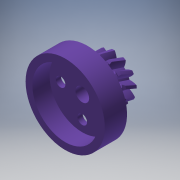
# Autodesk Inventor part: Stirnzahnrad2
Saved by Autodesk Inventor 2019.1 (Build 231200000, 200)
## iProperties
Created: 2019-01-01
Part Number: Stirnzahnrad2
Material: Steel
Document SubType Name: Modeling
Designer: JochenAlt
Categories: <?xml version="1.0" encoding="UTF-16"?> <MemberInstance><Categories><FamilyTemplate><FamilyTemplateParameter ValueType="xs:double" Id="1" ObjectReferenceKey="da_z" ObjectType="kUserParameterObject"/><FamilyTemplateParameter ValueType="xs:double" Id="2" ObjectReferenceKey="da_b" ObjectType="kUserParameterObject"/><FamilyTemplateParameter ValueType="xs:double" Id="3" ObjectReferenceKey="da_beta" ObjectType="kUserParameterObject"/><FamilyTemplateParameter ValueType="xs:double" Id="4" ObjectReferenceKey="da_da" ObjectType="kUserParameterObject"/><FamilyTemplateParameter ValueType="xs:double" Id="5" ObjectReferenceKey="da_aw" ObjectType="kUserParameterObject"/></FamilyTemplate><ParamToTemplateMap><ParamToTemplate CategoryParameter="//CategoryParameter[@InternalName='046C89C9-8512-4d59-83FE-43B91F4F132A']" TemplateParameter="1"/><ParamToTemplate CategoryParameter="//CategoryParameter[@InternalName='2552DF32-E462-4b46-AEBF-C6C7768E72AC']" TemplateParameter="2"/><ParamToTemplate CategoryParameter="//CategoryParameter[@InternalName='C9EE641D-15FC-4fae-A226-E94C4372FDD7']" TemplateParameter="3"/><ParamToTemplate><ParamToTemplate CategoryParameter="//CategoryParameter[@InternalName='00B6519A-459B-49c7-AD84-2E56D39A5744']" ConstantValue="-0.200000"/></ParamToTemplate><ParamToTemplate><ParamToTemplate CategoryParameter="//CategoryParameter[@InternalName='04B31F0E-C7A6-4894-AA32-9629BEFACF47']" ConstantValue="1.000000"/></ParamToTemplate><ParamToTemplate><ParamToTemplate CategoryParameter="//CategoryParameter[@InternalName='43CBEC2E-7847-49e7-A936-2F7889FCB2D9']" ConstantValue="0.250000"/></ParamToTemplate><ParamToTemplate><ParamToTemplate CategoryParameter="//CategoryParameter[@InternalName='B1EFC894-105D-4ebd-86BF-FA20ED196853']" ConstantValue="0.350000"/></ParamToTemplate><ParamToTemplate><ParamToTemplate CategoryParameter="//CategoryParameter[@InternalName='51175063-3D10-4879-93E8-6246FE8B403D']" ConstantValue="2060000000.000000"/></ParamToTemplate><ParamToTemplate><ParamToTemplate CategoryParameter="//CategoryParameter[@InternalName='A3A52E27-4454-46a9-B0BD-C932399B70AF']" ConstantValue="0.300000"/></ParamToTemplate><ParamToTemplate><ParamToTemplate CategoryParameter="//CategoryParameter[@InternalName='91B76062-C214-41d9-B1B9-14D2AB99603D']" ConstantValue="0.090000"/></ParamToTemplate><ParamToTemplate><ParamToTemplate CategoryParameter="//CategoryParameter[@InternalName='374E806E-8B8A-4dda-A9AA-1039D6500AD2']" ConstantValue="11.111111"/></ParamToTemplate><ParamToTemplate><ParamToTemplate CategoryParameter="//CategoryParameter[@InternalName='2D373A89-B862-43d6-8D0B-0CBF12AB9F6C']" ConstantValue="0.349066"/></ParamToTemplate><ParamToTemplate CategoryParameter="//CategoryParameter[@InternalName='37777632-D6A2-4fac-9D53-DB8ACD95C989']" TemplateParameter="4"/><ParamToTemplate CategoryParameter="//CategoryParameter[@InternalName='FD1017F1-B727-4f7e-9707-0F86F1FF9423']" TemplateParameter="5"/><ParamToTemplate><ParamToTemplate CategoryParameter="//CategoryParameter[@InternalName='9E1B4470-B2D3-4ff1-B813-535BB4CDF51A']" ConstantValue="3520000.000000"/></ParamToTemplate><ParamToTemplate><ParamToTemplate CategoryParameter="//CategoryParameter[@InternalName='F8452263-BFF6-458c-9FB1-07C4B99E95CD']" ConstantValue="11400000.000000"/></ParamToTemplate><ParamToTemplate><ParamToTemplate CategoryParameter="//CategoryParameter[@InternalName='3E3BB259-FD49-497f-8171-6EBC954A3479']" ConstantValue="2.000000"/></ParamToTemplate></ParamToTemplateMap><Category DisplayName="Gear" InternalName="DC85795E-93AB-48d5-8EEE-5A27447B64BD" Mnemonic="Gear"><CategoryParameter DisplayName="z" InternalName="046C89C9-8512-4d59-83FE-43B91F4F132A" Mnemonic="z"/><CategoryParameter DisplayName="b" InternalName="2552DF32-E462-4b46-AEBF-C6C7768E72AC" Mnemonic="b"/><CategoryParameter DisplayName="||b|" InternalName="C9EE641D-15FC-4fae-A226-E94C4372FDD7" Mnemonic="beta"/><CategoryParameter DisplayName="x" InternalName="00B6519A-459B-49c7-AD84-2E56D39A5744" Mnemonic="x"/><CategoryParameter DisplayName="a*" InternalName="04B31F0E-C7A6-4894-AA32-9629BEFACF47" Mnemonic="a"/><CategoryParameter DisplayName="c*" InternalName="43CBEC2E-7847-49e7-A936-2F7889FCB2D9" Mnemonic="c"/><CategoryParameter DisplayName="r|.f|*" InternalName="B1EFC894-105D-4ebd-86BF-FA20ED196853" Mnemonic="rf"/><CategoryParameter DisplayName="E" InternalName="51175063-3D10-4879-93E8-6246FE8B403D" Mnemonic="E"/><CategoryParameter DisplayName="||m|" InternalName="A3A52E27-4454-46a9-B0BD-C932399B70AF" Mnemonic="mi"/><Category DisplayName="SpurGear" InternalName="26C5A22E-A91E-4dfd-A3B3-23CCAFAE1764" Mnemonic="SpurGear"><CategoryParameter DisplayName="m" InternalName="91B76062-C214-41d9-B1B9-14D2AB99603D" Mnemonic="m"/><CategoryParameter DisplayName="P" InternalName="374E806E-8B8A-4dda-A9AA-1039D6500AD2" Mnemonic="PP"/><CategoryParameter DisplayName="||a|" InternalName="2D373A89-B862-43d6-8D0B-0CBF12AB9F6C" Mnemonic="alpha"/><CategoryParameter DisplayName="d|.a|" InternalName="37777632-D6A2-4fac-9D53-DB8ACD95C989" Mnemonic="da"/><CategoryParameter DisplayName="a|.w|" InternalName="FD1017F1-B727-4f7e-9707-0F86F1FF9423" Mnemonic="aw"/><CategoryParameter DisplayName="||s||.Flim|" InternalName="9E1B4470-B2D3-4ff1-B813-535BB4CDF51A" Mnemonic="sFlim"/><CategoryParameter DisplayName="||s||.Hlim|" InternalName="F8452263-BFF6-458c-9FB1-07C4B99E95CD" Mnemonic="sHlim"/><CategoryParameter DisplayName="Typ" InternalName="3E3BB259-FD49-497f-8171-6EBC954A3479" Mnemonic="type"/></Category></Category></Categories></MemberInstance>
Density: 1 g/cm^3
Appearance: Steel
CustomPartVersion: 1
Author: JochenAlt
Autodesk Inventor part; units mm, degrees
ref_plane "YZ Plane" through (0, 0, 0) normal (1, 0, 0) x (0, 1, 0)
ref_plane "XZ Plane" through (0, 0, 0) normal (0, 1, 0) x (-1, 0, 0)
ref_plane "XY Plane" through (0, 0, 0) normal (0, 0, 1) x (1, 0, 0)
sketch "Sketch1" plane through (0, 0, 0) normal (0, 0, 1) x (1, 0, 0)
  circle A0 centre (0, 0) radius 6.4343
  dimension "d0" = 12.8686
  constraints: 1 centre point
  measures "d0" diameter of A0
extrude "Extrusion1" add sketch "Sketch1" along normal blind 4.5
ref_plane "Work Plane2" through (0, 0, 2.25) normal (0, 0, 1) x (1, 0, 0)
ref_plane "Work Plane8" through (0, 0, 0) normal (0.9659258, 0.258819, 0) x (0, 0, 1)
ref_plane "Work Plane9" through (0, 0, 0) normal (1, 0, 0) x (0, 1, 0)
spur gear teeth "Stirnzahnrad" teeth 12 pitch diameter 11.4931 tip diameter 12.8686 root diameter 8.8831 face width 4.5 helix angle 20 hand right start plane through (0, 0, 0) normal (0, 0, -1) x (-1, 0, 0)
sketch "Skizze3" plane through (0, 0, 4.5) normal (0, 0, 1) x (1, 0, 0)
  circle A0 centre (0, 0) radius 5.9343
  circle A1 centre (0, 0) radius 6.4343
  circle A2 centre (0, 0) radius 2
  circle A3 centre (0, 0) radius 3.6
  circle A4 centre (0, 0) radius 3.1
  point P0 (1.4014, -6.2798)
  dimension "d57" = 0.5
  dimension "d59" = 4
  dimension "d78" = 7.2
  dimension "d81" = 0.5
  constraints: 5 coincident, 4 centre point, 3 other
  measures "d59" diameter of A2
  measures "d78" diameter of A3
  measures "d81" radial gap between concentric circles of A3 A4
mirror "Spiegeln1" about plane through (0, 0, 4.5) normal (0, 0, 1)
extrude "Extrusion12" cut sketch "Skizze3" along normal through all both and the other way through all contours A2
extrude "Extrusion13" cut sketch "Skizze3" along normal blind 3 from surface at -4.5 contours A3 | A4
extrude "Extrusion14" cut sketch "Skizze3" along normal blind 0.5 from surface at -1.5 contours A4
extrude "Extrusion2" add sketch "Skizze3" along normal mid plane 1 separate body contours A1
chamfer "Fase3" distance 0.5 angle 45 2 edges at (-5.9343, 0, 4) (-5.9343, 0, 5)
combine bodies "Kombinieren2" operation type subtract main body 1 bodies to subtract 2
sketch "Skizze6" plane through (0, 0, 0) normal (0, 0, 1) x (1, 0, 0)
  circle A0 centre (0, 0) radius 6.4343
  arc A1 (0.4208, 6.4205) -> (-0.4208, 6.4205) centre (0, 0) ccw projected
  constraints: 1 coincident, 3 other
extrude "Extrusion7" cut sketch "Skizze6" along normal blind 1 from surface at 0 bodies 1
sketch "Skizze4" plane through (0, 0, 9) normal (0, 0, 1) x (-1, 0, 0)
  circle A0 centre (0, 0) radius 2
  circle A1 centre (0, 0) radius 9.6
  circle A2 centre (0, 0) radius 6.35 construction
  circle A3 centre (6.35, 0) radius 1.4
  circle A4 centre (-6.35, 0) radius 1.4
  circle A5 centre (0, 6.35) radius 1.4
  circle A6 centre (0, -6.35) radius 1.4
  circle A7 centre (0, 0) radius 11.6
  line L0 (0, -16.24) -> (0, 16.24) construction
  line L1 (16.24, 0) -> (-16.24, 0) construction
  circle A8 centre (0, 0) radius 4.4416
  point P0 (2.9285, 3.3393)
  point P1 (2.9285, 3.3393)
  dimension "d65" = 19.2
  dimension "d66" = 12.7
  dimension "d67" = 2.8
  dimension "d68" = 4
  dimension "d69" = 2
  constraints: 8 centre point, 8 coincident, 4 point on circle, 4 point on line, 3 equal radius, 3 other
  measures "d65" diameter of A1
  measures "d66" diameter of A2
  measures "d67" diameter of A3
  measures "d68" diameter of A0
  measures "d69" radial gap between concentric circles of A1 A7
extrude "Extrusion4" add sketch "Skizze4" along normal blind 1.5 from surface at 0 contours A1 | A7 | A8 bodies 1
extrude "Extrusion5" add sketch "Skizze4" along normal blind 6.5 contours A7 bodies 1
equation "\"d0\" = da_da"
equation "\"d1\" = da_b"
equation "\"d16\" = da_aw"
equation "\"d43\" = da_aw"
equation "\"d46\" = da_aw"
equation "\"da_da\" = 12.868638"
equation "\"da_b\" = 4.5"
equation "\"da_aw\" = 16.847439"
body "Solid1"
